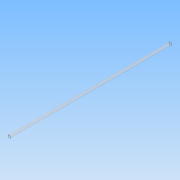
# Autodesk Inventor part: Top_End Pipe 1
Saved by Autodesk Inventor 2018.1 (Build 221171000, 171)
## iProperties
Created: 2019-03-21
Part Number: Top_End Pipe 1
Material: PMMA Plastic
Document SubType Name: Modeling
Designer: James
Density: 1.188 g/cm^3
Appearance: Polycarbonate - Clear
Author: James
Autodesk Inventor part; units mm, degrees
ref_plane "YZ Plane" through (0, 0, 0) normal (1, 0, 0) x (0, 1, 0)
ref_plane "XZ Plane" through (0, 0, 0) normal (0, 1, 0) x (-1, 0, 0)
ref_plane "XY Plane" through (0, 0, 0) normal (0, 0, 1) x (1, 0, 0)
sketch "Sketch1" plane through (0, 0, 0) normal (0, 1, 0) x (-1, 0, 0)
  circle A0 centre (0, 0) radius 23
  circle A1 centre (0, 0) radius 20
  dimension "d0" = 3
  dimension "d1" = 40
  constraints: 2 centre point, 2 coincident
  measures "d0" radial gap between concentric circles of A0 A1
  measures "d1" diameter of A1
extrude "Extrusion1" add sketch "Sketch1" along normal blind 2680.4
sketch "Sketch2" plane through (0, 0, 0) normal (0, 0, 1) x (1, 0, 0)
  line L0 (23, 2680.4) -> (-23, 2680.4) projected
  point P0 (0, 0)
  point P1 (0, 2673.4)
  point P2 (0, 2680.4)
  dimension "d4" = 7
  constraints: 1 midpoint, 1 vertical alignment
  measures "d4" distance from line of L0 point (0, 2673.4)
hole "Hole1" [suppressed]
sketch3d "3D Sketch1"
sketch "Sketch3" plane through (0, 0, 0) normal (0, -1, 0) x (1, 0, 0)
  circle A0 centre (0, 0) radius 20 projected
  circle A1 centre (0, 0) radius 23 projected
sweep "Sweep1" [suppressed]
sketch "Sketch4" plane through (162.5, -96, -92.5) normal (0, 0, -1) x (-1, 0, 0)
  circle A0 centre (0, 0) radius 23 projected
  point P0 (162.5, 96)
  point P1 (-19.7108, -3.389)
  point P2 (-22.6674, -3.8973)
  constraints: 2 other
extrude "Extrusion2" [suppressed]
sketch "Sketch5" plane through (0, 0, 0) normal (0, -1, 0) x (1, 0, 0)
  circle A0 centre (0, 0) radius 20 projected
  circle A1 centre (0, 0) radius 23 projected
sketch3d "3D Sketch2"
sweep "Sweep2" [suppressed]
sketch "Sketch6" plane through (0, -160, 405) normal (0, -1, 0) x (1, 0, 0)
  circle A0 centre (0, 0) radius 23 projected
  point P0 (0, -405)
  point P1 (20, 0)
  point P2 (23, 0)
  constraints: 1 horizontal alignment, 1 other
extrude "Extrusion3" [suppressed]
sketch "Sketch7" plane through (0, 0, 0) normal (1, 0, 0) x (0, 1, 0)
  line L0 (0, 23) -> (0, -23) projected
  line L1 (2680.4, -23) -> (2680.4, 23) projected
  point P0 (0, 0)
  point P1 (5, 0)
  point P2 (2675.4, 0)
  dimension "d35" = 5
  dimension "d36" = 5
  constraints: 2 horizontal alignment
  measures "d35" distance from line of point (5, 0) L0
  measures "d36" distance from line of point (2675.4, 0) L1
hole "Hole2" at (0, 5, 0) at (0, 2675.4, 0) direction (-1, 0, 0) diameter 4.5 end through all
body "Solid1"
